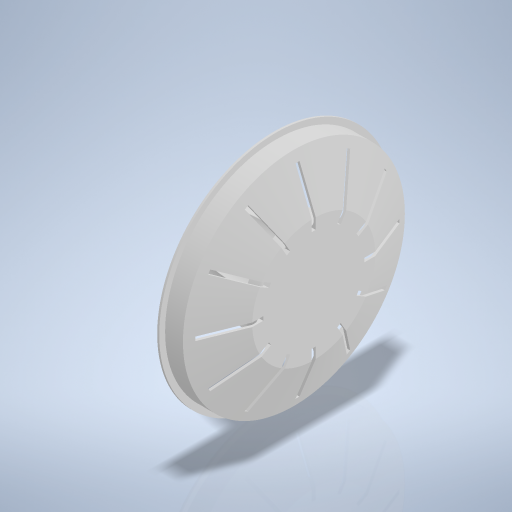
# Autodesk Inventor part: sieve
Saved by Autodesk Inventor 2024 (Build 280153000, 153)
## iProperties
Created: 2024-04-26
Part Number: sieve
Material: Generisch
Document SubType Name: Modeling
Designer: ffogue
Density: 1 g/cm^3
Appearance: Vorgabe
Author: ffogue
Autodesk Inventor part; units mm, degrees
sketch "Skizze1" plane through (0, 0, 0) normal (0, 1, 0) x (-1, 0, 0)
  line L0 (0, -125) -> (0, -155)
  line L1 (0, -155) -> (50, -280)
  line L2 (50, -280) -> (95, -280)
  line L3 (95, -280) -> (95, -295)
  line L4 (95, -295) -> (100, -295)
  line L5 (100, -295) -> (100, -275)
  line L6 (100, -275) -> (55, -275)
  line L7 (55, -275) -> (5, -150)
  line L8 (5, -150) -> (5, -125)
  line L9 (0, -125) -> (5, -125)
  line L10 (0, 0) -> (280, 0)
  point P0 (0, -155)
  dimension "d1" = 20
  dimension "d2" = 30
  dimension "d5" = 5
  dimension "d6" = 5
  dimension "d7" = 150
  dimension "d8" = 50
  dimension "d10" = 100
  dimension "d29" = 125
  dimension "d39" = 280
  constraints: 22 end point, 6 perpendicular, 3 parallel, 2 horizontal, 1 vertical, 1 vertical alignment
  measures "d1" distance between parallel lines of L4 L6
  measures "d2" distance of L0.start L0.end
  measures "d5" distance between parallel lines of L2 L6
  measures "d6" distance between parallel lines of L3 L5
  measures "d7" distance from line of L0.start L6
  measures "d8" horizontal distance of L1.end L0.end
  measures "d10" distance from line of L5 L0.end
  measures "d29" distance of L10.start L0.start
  measures "d39" distance of L10.start L10.end
revolve "Umdrehung4" add sketch "Skizze1" angle 360 about axis through (0, 0, 0) along (-1, 0, 0)
sketch "Skizze2" plane through (0, 0, 0) normal (1, 0, 0) x (0, 0, -1)
  circle A0 centre (0, 0) radius 125 projected
extrude "Extrusion1" add sketch "Skizze2" against normal blind 50
fillet "Rundung1" radius 20 1 edges at (-5, 0, 125)
ref_plane "Arbeitsebene1" through (-100, 0, 0) normal (-1, 0, 0) x (0, 0, 1)
sketch "Skizze3" plane through (-100, 0, 0) normal (-1, 0, 0) x (0, 0, 1)
  circle A0 centre (0, 0) radius 145 projected
  circle A1 centre (0, 0) radius 125 projected
  line L0 (-257.4551, 5) -> (-127.4551, 5)
  line L1 (-127.4551, 5) -> (-127.4551, -5)
  line L2 (-127.4551, -5) -> (-257.4551, -5)
  line L3 (-257.4551, -5) -> (-257.4551, 5)
  line L4 (0, 0) -> (-436.9382, 0) construction
  line L5 (-220.4626, 133.0577) -> (-107.8793, 68.0577)
  line L6 (-112.8793, 59.3974) -> (-225.4626, 124.3974)
  line L7 (-107.8793, 68.0577) -> (-112.8793, 59.3974)
  line L8 (-225.4626, 124.3974) -> (-220.4626, 133.0577)
  line L9 (-124.3974, 225.4626) -> (-59.3974, 112.8793)
  line L10 (-68.0577, 107.8793) -> (-133.0577, 220.4626)
  line L11 (-59.3974, 112.8793) -> (-68.0577, 107.8793)
  line L12 (-133.0577, 220.4626) -> (-124.3974, 225.4626)
  line L13 (5, 257.4551) -> (5, 127.4551)
  line L14 (-5, 127.4551) -> (-5, 257.4551)
  line L15 (5, 127.4551) -> (-5, 127.4551)
  line L16 (-5, 257.4551) -> (5, 257.4551)
  line L17 (133.0577, 220.4626) -> (68.0577, 107.8793)
  line L18 (59.3974, 112.8793) -> (124.3974, 225.4626)
  line L19 (68.0577, 107.8793) -> (59.3974, 112.8793)
  line L20 (124.3974, 225.4626) -> (133.0577, 220.4626)
  line L21 (225.4626, 124.3974) -> (112.8793, 59.3974)
  line L22 (107.8793, 68.0577) -> (220.4626, 133.0577)
  line L23 (112.8793, 59.3974) -> (107.8793, 68.0577)
  line L24 (220.4626, 133.0577) -> (225.4626, 124.3974)
  line L25 (257.4551, -5) -> (127.4551, -5)
  line L26 (127.4551, 5) -> (257.4551, 5)
  line L27 (127.4551, -5) -> (127.4551, 5)
  line L28 (257.4551, 5) -> (257.4551, -5)
  line L29 (220.4626, -133.0577) -> (107.8793, -68.0577)
  line L30 (112.8793, -59.3974) -> (225.4626, -124.3974)
  line L31 (107.8793, -68.0577) -> (112.8793, -59.3974)
  line L32 (225.4626, -124.3974) -> (220.4626, -133.0577)
  line L33 (124.3974, -225.4626) -> (59.3974, -112.8793)
  line L34 (68.0577, -107.8793) -> (133.0577, -220.4626)
  line L35 (59.3974, -112.8793) -> (68.0577, -107.8793)
  line L36 (133.0577, -220.4626) -> (124.3974, -225.4626)
  line L37 (-5, -257.4551) -> (-5, -127.4551)
  line L38 (5, -127.4551) -> (5, -257.4551)
  line L39 (-5, -127.4551) -> (5, -127.4551)
  line L40 (5, -257.4551) -> (-5, -257.4551)
  line L41 (-133.0577, -220.4626) -> (-68.0577, -107.8793)
  line L42 (-59.3974, -112.8793) -> (-124.3974, -225.4626)
  line L43 (-68.0577, -107.8793) -> (-59.3974, -112.8793)
  line L44 (-124.3974, -225.4626) -> (-133.0577, -220.4626)
  line L45 (-225.4626, -124.3974) -> (-112.8793, -59.3974)
  line L46 (-107.8793, -68.0577) -> (-220.4626, -133.0577)
  line L47 (-112.8793, -59.3974) -> (-107.8793, -68.0577)
  line L48 (-220.4626, -133.0577) -> (-225.4626, -124.3974)
  dimension "d47" = 130
  dimension "d48" = 127.4551
  dimension "d49" = 10
  dimension "d63" = 360
  constraints: 98 end point, 2 horizontal, 2 parallel, 1 perpendicular, 98 other
  measures "d47" distance between parallel lines of L1 L3
  measures "d48" distance from line of point (0, 0) L1
  measures "d49" distance between parallel lines of L2 L0
extrude "Extrusion4" cut sketch "Skizze3" against normal up to surface (100 mm away) contours A0 L25 L27 L26 | A0 L26 L28 L25 | L21 L23 L22 A0 | A0 L22 L24 L21 | L30 L32 L29 A0 | A0 L29 L31 L30 | L17 L19 L18 A0 | A0 L18 L20 L17 | L34 L36 L33 A0 | A0 L33 L35 L34 | L13 L15 L14 A0 | A0 L14 L16 L13 | L38 L40 L37 A0 | A0 L37 L39 L38 | L9 L11 L10 A0 | A0 L10 L12 L9 | L42 L44 L41 A0 | A0 L41 L43 L42 | L5 L7 L6 A0 | A0 L6 L8 L5 | L46 L48 L45 A0 | A0 L45 L47 L46 | L0 L1 L2 A0 | A0 L2 L3 L0
sketch "Skizze6" plane through (-50, 0, 0) normal (-1, 0, 0) x (0, 0, 1)
  circle A0 centre (0, 0) radius 125 projected
extrude "Extrusion5" add sketch "Skizze6" along normal blind 230
ref_plane "Arbeitsebene4" through (0, 0, 0) normal (0, 0, 1) x (1, 0, 0)
sketch "Skizze7" plane through (0, 0, 0) normal (0, 0, 1) x (1, 0, 0)
  line L0 (0, 0) -> (-329.521, 0)
  line L1 (-280, 125) -> (-280, -125) projected
  line L2 (-25, -125) -> (-280, -125) projected
  line L3 (-50, -125) -> (-50, 125) construction
  line L4 (-25, 125) -> (-280, 125) projected
  line L5 (-50, 125) -> (-50, 0)
  arc A0 (-191.249, 104.6339) -> (-280, 0) centre (-155.9368, -15.2745) ccw
  arc A1 (-50, 125) -> (-191.249, 104.6339) centre (-50, -375) ccw
  dimension "d78" = 230
  dimension "d96" = 125
  dimension "d97" = 500
  constraints: 6 end point, 4 point on circle, 2 centre point, 2 midpoint, 2 point on line, 2 tangent, 1 horizontal, 1 vertical
  measures "d78" distance between parallel lines of L3 L1
  measures "d96" radius of A0
  measures "d97" radius of A1
revolve "Umdrehung5" cut sketch "Skizze7" angle 360 about axis through (0, 0, 0) along (-1, 0, 0) contours L1 L4 A1 A0
ref_plane "Arbeitsebene5" through (-50, 0, 0) normal (-1, 0, 0) x (0, -1, 0)
ref_plane "Arbeitsebene7" through (-60, 0, 0) normal (-1, 0, 0) x (0, -1, 0)
sketch "Skizze10" plane through (-60, 0, 0) normal (-1, 0, 0) x (0, -1, 0)
  arc A0 (124.0462, -8.9493) -> (124.0462, 8.9493) centre (0, 0) ccw projected
  arc A1 (124.676, 8.9942) -> (124.676, -8.9942) centre (0, 0) ccw projected
  circle A2 centre (124.3686, 0) radius 15
  point P0 (124.097, 14.9975)
  point P1 (124.097, -14.9975)
  point P2 (123.9666, 9.9919)
  point P3 (123.9666, -9.9919)
  dimension "d89" = 30
  constraints: 1 centre point, 1 point on circle, 2 other
  measures "d89" diameter of A2
ref_plane "Arbeitsebene8" through (0, 0, 0) normal (0, 0, 1) x (1, 0, 0)
ref_plane "Arbeitsebene9" through (-60, 0, 0) normal (-1, 0, 0) x (0, -1, 0)
sketch "Skizze13" plane through (-60, 0, 0) normal (-1, 0, 0) x (0, -1, 0)
  circle A0 centre (150, 0) radius 42.5
  point P0 (0, 0)
  point P1 (125, 0)
  dimension "d105" = 150
  dimension "d106" = 85
  constraints: 1 centre point, 1 horizontal alignment
  measures "d105" distance of point (0, 0) A0.centre
  measures "d106" diameter of A0
sketch "Skizze14" plane through (0, 0, 0) normal (0, 0, 1) x (1, 0, 0)
  arc A0 (-191.249, -104.6339) -> (-50, -125) centre (-50, 375) ccw projected
  arc A1 (-280, 0) -> (-191.249, -104.6339) centre (-155.9368, 15.2745) ccw projected
  point P0 (0, 0)
sweep "Sweeping3" cut profiles "Skizze13" path "Skizze14"
pattern_circular "Runde Anordnung3" count 12 over 360 about axis through (-77.5, 0, 0) along (-1, 0, 0) of "Sweeping3"
fillet "Rundung2" radius 2 24 edges at (-86.8985, 119.1591, -32.9714) (-86.8985, 119.6806, -31.0255) (-86.8985, 119.6806, 31.0255) (-86.8985, 119.1591, 32.9714) (-86.8985, 88.1337, 86.7091) (-86.8985, 86.7091, 88.1337) (-86.8985, 32.9714, 119.1591) (-86.8985, 31.0255, 119.6806) (-86.8985, -32.9714, 119.1591) (-86.8985, -86.7091, 88.1337) (-86.8985, -88.1337, 86.7091) (-86.8985, -119.1591, 32.9714) (-86.8985, -119.6806, -31.0255) (-86.8985, -119.6806, 31.0255) (-86.8985, -119.1591, -32.9714) (-86.8985, -88.1337, -86.7091) (-86.8985, -86.7091, -88.1337) (-86.8985, -32.9714, -119.1591) (-86.8985, 31.0255, -119.6806) (-86.8985, 32.9714, -119.1591) (-86.8985, 86.7091, -88.1337) (-86.8985, 88.1337, -86.7091) (-86.8985, -31.0255, -119.6806) (-86.8985, -31.0255, 119.6806)
equation "\"d5\" = d6"
